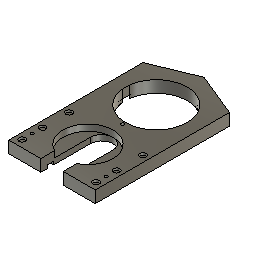
R7 Dust Boot v1 (Autodesk Fusion 360 design; units mm, degrees)
Autodesk Fusion 360 part; units mm, degrees
sketch "Sketch1" plane through (0, 0, 0) normal (0, 0, 1) x (1, 0, 0)
  line L0 (0, 0) -> (0, 152.4) construction
  line L1 (0, 152.4) -> (-43.3705, 134.62)
  line L2 (-43.3705, 134.62) -> (-43.3705, 0)
  line L3 (-43.3705, 0) -> (0, 0)
  line L4 (-11.2014, 49.7586) -> (-11.2014, 0)
  arc A0 (0, 60.96) -> (-11.2014, 49.7586) centre (0, 49.7586) ccw
  arc A1 (0, 60.96) -> (-11.2014, 13.7311) centre (0, 36.0172) ccw
  line L5 (0, 145.5371) -> (-37.0205, 130.3603)
  line L6 (-37.0205, 130.3603) -> (-37.0205, 6.35)
  line L7 (-37.0205, 6.35) -> (-11.2014, 6.35)
  line L8 (0, 138.6742) -> (-30.6705, 126.1007)
  line L9 (-30.6705, 126.1007) -> (-30.6705, 12.7)
  line L10 (-30.6705, 12.7) -> (-11.2014, 12.7)
  line L11 (30.6705, 12.7) -> (11.2014, 12.7)
  line L12 (37.0205, 130.3603) -> (37.0205, 6.35)
  line L13 (0, 145.5371) -> (37.0205, 130.3603)
  line L14 (0, 138.6742) -> (30.6705, 126.1007)
  line L15 (37.0205, 6.35) -> (11.2014, 6.35)
  arc A2 (11.2014, 49.7586) -> (0, 60.96) centre (0, 49.7586) ccw
  line L16 (11.2014, 49.7586) -> (11.2014, 0)
  line L17 (43.3705, 134.62) -> (43.3705, 0)
  line L18 (30.6705, 126.1007) -> (30.6705, 12.7)
  arc A3 (11.2014, 13.7311) -> (0, 60.96) centre (0, 36.0172) ccw
  line L19 (43.3705, 0) -> (0, 0)
  line L20 (0, 152.4) -> (43.3705, 134.62)
  circle A4 centre (0, 104.6382) radius 30.861
  point P0 (0, 60.96)
  point P1 (0, 60.96)
  point P2 (0, 135.4992)
  dimension "d1" = 152.4
  dimension "d2" = 43.3705
  dimension "d3" = 134.62
  dimension "d4" = 49.8856
  dimension "d5" = 22.4028
  dimension "d6" = 60.96
  dimension "d9" = 6.35
  dimension "d10" = 6.35
  dimension "d11" = 6.35
  dimension "d12" = 6.35
  dimension "d13" = 6.35
  dimension "d14" = 6.35
  dimension "d22" = 61.722
  dimension "d23" = 3.175
  constraint coincident L0.start L3.end
  constraint vertical L0
  constraint parallel L0 L2
  constraint perpendicular L0 L3
  constraint coincident L0 A1.centre
  constraint coincident L0 A0.centre
  constraint coincident L3 L4.end
  constraint tangent L4 A0
  constraint perpendicular L3 L4
  constraint coincident L0 P1
  constraint coincident P1 A0
  constraint coincident P1 P0
  constraint coincident L4 A1.end
  constraint parallel L1 L8
  constraint parallel L2 L9
  constraint parallel L3 L10
  constraint coincident L4 L10.end
  constraint parallel L1 L5
  constraint parallel L2 L6
  constraint parallel L3 L7
  constraint coincident L4 L7.end
  constraint coincident L0 L5.start
  constraint coincident L0 L8.start
  constraint symmetric L3.end L0 L19.end
  constraint symmetric L1.start L0 L20.start
  constraint symmetric L0 L1.end L17.start
  constraint symmetric L0 L2.end L17.end
  constraint symmetric L0 L3.end L19.end
  constraint symmetric L0 L4.start A2.start
  constraint symmetric L0 L4.end L16.end
  constraint symmetric L0 P1 P0
  constraint symmetric L0 A0 A2
  constraint symmetric L0 A1 A3
  constraint symmetric L0 A1.end A3.start
  constraint symmetric L0 L5.end L12.start
  constraint symmetric L0 L6.end L12.end
  constraint symmetric L0 L8.end L14.end
  constraint symmetric L0 L9.end L11.start
  constraint symmetric L0 L10.end L11.end
  constraint symmetric L0 L7.end L15.end
  constraint symmetric L0 L5.start L13.start
  constraint symmetric L0 L8.start L14.start
  constraint coincident L0 A4.centre
  constraint coincident A4 P2
  constraint coincident L0 P2
  measures "d1" distance of L0.start L0.end
  measures "d2" distance of L2.end L0.start
  measures "d3" distance of L1.end L2.end
  measures "d4" diameter of A1
  measures "d5" diameter of A0
  measures "d6" distance of L0.start P1
  measures "d9" distance of L1 L5
  measures "d10" distance of L5 L8
  measures "d11" distance of L2 L6
  measures "d12" distance of L6 L9
  measures "d13" distance of L7 L10
  measures "d14" distance of L3 L7
  measures "d22" diameter of A4
  measures "d23" distance of L8.start P2
extrude "Extrude1" add sketch "Sketch1" along normal blind 11.9126 contours L1 L2 L3 L4 L5 L6 L7 L12 L13 L15 L16 L17 L19 L20 | L4 L5 L6 L7 L8 L9 L10 L11 L12 L13 L14 L15 L16 L18 A4 | L4 A1 L9 L10 L11 L16 L18 A3 A4 | L4 A0 A1 | A2 L16 A3 | L9 A4 | L18 A4 | L8 L9 L14 L18 A4
extrude "Extrude2" cut sketch "Sketch1" against normal blind 6.35 from surface at 11.9126 contours L4 A0 A1 | A2 L16 A3
extrude "Extrude3" cut sketch "Sketch1" along normal blind 3.175 contours L4 L5 L6 L7 L8 L9 L10 L11 L12 L13 L14 L15 L16 L18 A4 | L9 A4 | L18 A4
sketch "Sketch2" plane through (0, 0, 11.9126) normal (0, 0, 1) x (-1, 0, 0)
  line L0 (30.6705, -101.2145) -> (30.6705, -108.0619)
  arc A0 (-30.6705, -108.0619) -> (30.6705, -108.0619) centre (0, -104.6382) ccw
  line L1 (-30.6705, -108.0619) -> (-30.6705, -101.2145)
  arc A1 (30.6705, -101.2145) -> (-30.6705, -101.2145) centre (0, -104.6382) ccw
  arc A2 (-11.2014, -13.7311) -> (11.2014, -13.7311) centre (0, -36.0172) ccw
  line L2 (-11.2014, -13.7311) -> (-11.2014, 0)
  line L3 (-11.2014, 0) -> (-43.3705, 0)
  line L4 (-43.3705, 0) -> (-43.3705, -134.62)
  line L5 (-43.3705, -134.62) -> (0, -152.4)
  line L6 (0, -152.4) -> (43.3705, -134.62)
  line L7 (43.3705, -134.62) -> (43.3705, 0)
  line L8 (43.3705, 0) -> (11.2014, 0)
  line L9 (11.2014, 0) -> (11.2014, -13.7311)
  line L10 (0, -152.4) -> (0, 0) construction
  circle A3 centre (0, -71.12) radius 1.5748
  line L11 (37.1348, -17.2212) -> (-37.1348, -17.2212) construction
  circle A4 centre (37.1348, -17.2212) radius 1.5748
  circle A5 centre (-37.1348, -17.2212) radius 1.5748
  point P0 (0, -17.2212)
  dimension "d24" = 3.1496
  dimension "d25" = 74.2696
  dimension "d26" = 3.1496
  dimension "d27" = 3.1496
  dimension "d28" = 17.2212
  dimension "d30" = 71.12
  constraint coincident L5.end L6.start
  constraint coincident L10.end origin
  constraint coincident L10 A3.centre
  constraint perpendicular L2 L11
  constraint midpoint L11 P0
  constraint coincident L10 P0
  constraint coincident L11.start A4.centre
  constraint coincident L11.end A5.centre
  measures "d24" diameter of A3
  measures "d25" distance of L11.start L11.end
  measures "d26" diameter of A4
  measures "d27" diameter of A5
  measures "d28" distance of L10.end P0
  measures "d30" distance of L3 A3.centre
extrude "Extrude4" cut sketch "Sketch2" against normal blind 4.7625 contours A3 | A4 | A5
sketch "Sketch3" plane through (0, 0, 11.9126) normal (0, 0, 1) x (-1, 0, 0)
  circle A0 centre (0, -71.12) radius 1.5748
  circle A1 centre (-37.1348, -17.2212) radius 1.5748
  circle A2 centre (37.1348, -17.2212) radius 1.5748
  line L0 (30.6705, -101.2145) -> (30.6705, -108.0619)
  arc A3 (-30.6705, -108.0619) -> (30.6705, -108.0619) centre (0, -104.6382) ccw
  line L1 (-30.6705, -108.0619) -> (-30.6705, -101.2145)
  arc A4 (30.6705, -101.2145) -> (-30.6705, -101.2145) centre (0, -104.6382) ccw
  arc A5 (-11.2014, -13.7311) -> (11.2014, -13.7311) centre (0, -36.0172) ccw
  line L2 (-11.2014, -13.7311) -> (-11.2014, 0)
  line L3 (-11.2014, 0) -> (-43.3705, 0)
  line L4 (-43.3705, 0) -> (-43.3705, -134.62)
  line L5 (-43.3705, -134.62) -> (0, -152.4)
  line L6 (0, -152.4) -> (43.3705, -134.62)
  line L7 (43.3705, -134.62) -> (43.3705, 0)
  line L8 (43.3705, 0) -> (11.2014, 0)
  line L9 (11.2014, 0) -> (11.2014, -13.7311)
  line L10 (37.1348, 0) -> (37.1348, -137.1764) construction
  circle A6 centre (37.1348, -7.1374) radius 3.175
  circle A7 centre (37.1348, -27.6606) radius 3.175
  circle A8 centre (37.1348, -54.1782) radius 3.175
  line L11 (0, -152.4) -> (0, 0) construction
  circle A9 centre (-37.1348, -27.6606) radius 3.175
  circle A10 centre (-37.1348, -54.1782) radius 3.175
  circle A11 centre (-37.1348, -7.1374) radius 3.175
  dimension "d33" = 6.35
  dimension "d34" = 6.35
  dimension "d35" = 6.35
  dimension "d36" = 7.1374
  dimension "d37" = 20.5232
  dimension "d38" = 26.5176
  constraint coincident L8 L10.start
  constraint coincident L6 L10.end
  constraint perpendicular L8 L10
  constraint coincident A2.centre L10
  constraint coincident L10 A6.centre
  constraint coincident L10 A7.centre
  constraint coincident L10 A8.centre
  constraint coincident L5.end L6.start
  constraint coincident L11.end origin
  constraint symmetric A6 L11 A11
  constraint symmetric A7 L11 A9
  constraint symmetric A8 L11 A10
  measures "d33" diameter of A6
  measures "d34" diameter of A7
  measures "d35" diameter of A8
  measures "d36" distance of L10.start A6.centre
  measures "d37" distance of A6.centre A7.centre
  measures "d38" distance of A7.centre A8.centre
extrude "Extrude5" cut sketch "Sketch3" against normal blind 2.2098 contours A6 | A7 | A8 | A9 | A10 | A11
equation "d2 = 3.415 in / 2"
equation "d25 = 3.048 in - 0.124 in"
equation "d31 = ( -3 / 16 ) * 1 in"
